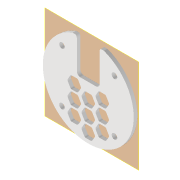
# Autodesk Inventor part: IM_Matchboxscope_base_xiao_lid
Saved by Autodesk Inventor 2022 (Build 260153000, 153)
## iProperties
Created: 2023-04-27
Part Number: IM_Matchboxscope_base_xiao_lid
Material: Generisch
Document SubType Name: Modeling
Designer: diederichbenedict
Density: 1 g/cm^3
Appearance: Vorgabe
Author: diederichbenedict
Autodesk Inventor part; units mm, degrees
ref_plane "YZ Plane" through (0, 0, 0) normal (1, 0, 0) x (0, 1, 0)
ref_plane "XZ Plane" through (0, 0, 0) normal (0, 1, 0) x (-1, 0, 0)
ref_plane "XY Plane" through (0, 0, 0) normal (0, 0, 1) x (1, 0, 0)
ref_plane "Arbeitsebene1" through (0, 0, 0) normal (0, 0, 1) x (1, 0, 0)
sketch "Skizze1" plane through (0, 0, 0) normal (0, 0, 1) x (1, 0, 0)
  line L0 (8.0712, 15) -> (38.0712, 15)
  line L1 (38.0712, 15) -> (38.0712, -15)
  line L2 (38.0712, -15) -> (8.0712, -15)
  line L3 (8.0712, -15) -> (8.0712, 15)
  line L4 (38.0712, 19) -> (8.0712, 19)
  line L5 (4.0712, 15) -> (4.0712, -15)
  line L6 (8.0712, -19) -> (38.0712, -19)
  line L7 (42.0712, -15) -> (42.0712, 15)
  arc A0 (8.0712, 19) -> (4.0712, 15) centre (8.0712, 15) ccw
  arc A1 (42.0712, 15) -> (38.0712, 19) centre (38.0712, 15) ccw
  arc A2 (38.0712, -19) -> (42.0712, -15) centre (38.0712, -15) ccw
  arc A3 (4.0712, -15) -> (8.0712, -19) centre (8.0712, -15) ccw
  line L8 (29.9712, -18.3074) -> (29.9712, -24.4) projected
  circle A4 centre (38.0712, -15) radius 1.4 projected
  circle A5 centre (38.0712, 15) radius 1.4 projected
  line L9 (39.5712, -24.4) -> (29.9712, -24.4) projected
  line L10 (39.5712, -21.1181) -> (39.5712, -24.4) projected
  line L11 (44.1893, -16.5) -> (39.5712, -21.1181) projected
  line L12 (47.4712, -16.5) -> (44.1893, -16.5) projected
  line L13 (47.4712, 16.5) -> (47.4712, -16.5) projected
  line L14 (44.1893, 16.5) -> (47.4712, 16.5) projected
  line L15 (39.5712, 21.1181) -> (44.1893, 16.5) projected
  line L16 (39.5712, 24.4) -> (39.5712, 21.1181) projected
  line L17 (31.5712, 24.4) -> (39.5712, 24.4) projected
  line L18 (31.5712, 4.0068) -> (31.5712, 24.4) projected
  arc A6 (32.7786, 1.7) -> (31.5712, 4.0068) centre (29.9712, 1.7) ccw projected
  line L19 (32.7786, 1.7) -> (32.7786, -15.5) projected
  arc A7 (29.9712, -18.3074) -> (32.7786, -15.5) centre (29.9712, -15.5) ccw projected
  arc A8 (16.5712, 25.149) -> (3.3138, -16.9) centre (23.0897, -0.0206) ccw
  circle A9 centre (23.0897, -0.0206) radius 26
  point P0 (0, 0)
  point P1 (36.5793, -24.4)
  point P2 (31.5712, 11.3758)
  point P3 (3.3138, -16.9)
  dimension "d0" = 4
  dimension "d1" = 4
  constraints: 16 end point, 10 point on circle, 8 tangent, 5 centre point, 4 parallel, 3 equal radius, 2 perpendicular, 1 coincident, 1 horizontal, 10 other
  measures "d0" distance between parallel lines of L0 L4
  measures "d1" radius of A0
extrude "Extrusion1" add sketch "Skizze1" along normal blind 2 contours L3 L2 L19 A7 L8 L6 A3 L5 A0 L4 L18 L0 | L0 L18 A6 L19 L2 L3 | L18 L4 A1 L7 A2 L6 L8 A7 L19 L2 A4 L1 A5 L0 | L0 A5 L1 A4 L2 L19 A6 L18 | A5 L1 L0 | L0 L1 A5 | L18 L17 A9 L13 L9 L8 L6 A2 L7 A1 L4 | L4 A0 L5 A3 L6 L8 L9 A9 A8 L17 L18 | A4 L1 L2 | L2 L1 A4 | A9 L13
ref_plane "Arbeitsebene2" through (0, 0, 0) normal (0, 0, 1) x (1, 0, 0)
sketch "Skizze2" plane through (0, 0, 2) normal (0, 0, 1) x (1, 0, 0)
  arc A0 (8.0712, 19) -> (4.0712, 15) centre (8.0712, 15) ccw projected
  line L0 (4.0712, 15) -> (4.0712, -15) projected
  arc A1 (4.0712, -15) -> (8.0712, -19) centre (8.0712, -15) ccw projected
  line L1 (8.0712, -19) -> (38.0712, -19) projected
  arc A2 (38.0712, -19) -> (42.0712, -15) centre (38.0712, -15) ccw projected
  line L2 (42.0712, -15) -> (42.0712, 15) projected
  arc A3 (42.0712, 15) -> (38.0712, 19) centre (38.0712, 15) ccw projected
  line L3 (38.0712, 19) -> (8.0712, 19) projected
  circle A4 centre (8.0712, 15) radius 1.4 projected
  circle A5 centre (38.0712, 15) radius 1.4 projected
  circle A6 centre (38.0712, -15) radius 1.4 projected
  circle A7 centre (8.0712, -15) radius 1.4 projected
  point P0 (0, 0)
hole "Bohrung1" at (8.0712, 15, 2) at (8.0712, -15, 2) at (38.0712, -15, 2) at (38.0712, 15, 2) direction (0, 0, -1) diameter 3.2 end through all
sketch "Skizze3" plane through (0, 0, 2) normal (0, 0, 1) x (1, 0, 0)
  circle A0 centre (23.0919, -0.0207) radius 4.25 projected
  arc A1 (30.2483, 24.4) -> (29.5712, 22.9) centre (31.5712, 22.9) ccw projected
  line L0 (39.5712, 24.4) -> (30.2483, 24.4) projected
  line L1 (39.5712, 21.1181) -> (39.5712, 24.4) projected
  line L2 (44.1893, 16.5) -> (39.5712, 21.1181) projected
  line L3 (47.4712, 16.5) -> (44.1893, 16.5) projected
  line L4 (47.4712, -16.5) -> (47.4712, 16.5) projected
  line L5 (44.1893, -16.5) -> (47.4712, -16.5) projected
  line L6 (39.5712, -21.1181) -> (44.1893, -16.5) projected
  line L7 (39.5712, -24.4) -> (39.5712, -21.1181) projected
  line L8 (6.6126, -24.4) -> (39.5712, -24.4) projected
  line L9 (6.6126, -21.1595) -> (6.6126, -24.4) projected
  line L10 (1.9531, -16.5) -> (6.6126, -21.1595) projected
  line L11 (-1.3288, -16.5) -> (1.9531, -16.5) projected
  line L12 (-1.3288, 16.5) -> (-1.3288, -16.5) projected
  line L13 (1.9531, 16.5) -> (-1.3288, 16.5) projected
  line L14 (6.5712, 21.1181) -> (1.9531, 16.5) projected
  line L15 (6.5712, 24.4) -> (6.5712, 21.1181) projected
  line L16 (15.894, 24.4) -> (6.5712, 24.4) projected
  arc A2 (16.5712, 22.9) -> (15.894, 24.4) centre (14.5712, 22.9) ccw projected
  line L17 (16.5712, 22.9) -> (16.5712, 6.5074) projected
  arc A3 (16.5712, 6.5074) -> (18.5712, 4.5074) centre (18.5712, 6.5074) ccw projected
  line L18 (18.5712, 4.5074) -> (27.5712, 4.5074) projected
  arc A4 (27.5712, 4.5074) -> (29.5712, 6.5074) centre (27.5712, 6.5074) ccw projected
  line L19 (29.5712, 6.5074) -> (29.5712, 22.9) projected
  circle A5 centre (38.0712, 15) radius 1.4 projected
  circle A6 centre (8.0712, -15) radius 1.4 projected
  circle A7 centre (38.0712, -15) radius 1.4 projected
  circle A8 centre (8.0712, 15) radius 1.4 projected
  line L20 (15.894, 24.4) -> (30.2483, 24.4)
  line L21 (6.5712, 24.4) -> (39.5712, 24.4)
  line L22 (39.5712, 24.4) -> (39.5712, 27.6612)
  line L23 (39.5712, 27.6612) -> (6.5712, 27.6612)
  line L24 (6.5712, 27.6612) -> (6.5712, 24.4)
  point P0 (0, 0)
  constraints: 10 end point, 2 horizontal, 2 parallel, 1 perpendicular
extrude "Extrusion2" cut sketch "Skizze3" against normal blind 10 contours L20 L16 L24 L23 L22 L0 | A1 L19 A4 L18 A3 L17 A2 L20
fillet "Rundung1" [suppressed]
sketch "Skizze4" plane through (0, 0, 2) normal (0, 0, 1) x (1, 0, 0)
  line L0 (32.0136, 24.4) -> (30.2483, 24.4) projected
  arc A0 (30.2483, 24.4) -> (29.5712, 22.9) centre (31.5712, 22.9) ccw projected
  line L1 (29.5712, 22.9) -> (29.5712, 6.5074) projected
  arc A1 (27.5712, 4.5074) -> (29.5712, 6.5074) centre (27.5712, 6.5074) ccw projected
  line L2 (27.5712, 4.5074) -> (18.5712, 4.5074) projected
  arc A2 (16.5712, 6.5074) -> (18.5712, 4.5074) centre (18.5712, 6.5074) ccw projected
  line L3 (16.5712, 6.5074) -> (16.5712, 22.9) projected
  arc A3 (16.5712, 22.9) -> (15.894, 24.4) centre (14.5712, 22.9) ccw projected
  line L4 (15.894, 24.4) -> (14.1659, 24.4) projected
  arc A4 (14.1659, 24.4) -> (32.0136, 24.4) centre (23.0897, -0.0206) ccw projected
  circle A5 centre (38.0712, 15) radius 1.6 projected
  circle A6 centre (8.0712, -15) radius 1.6 projected
  circle A7 centre (8.0712, 15) radius 1.6 projected
  circle A8 centre (38.0712, -15) radius 1.6 projected
  line L5 (19.3598, -3.9564) -> (20.7825, -1.4923)
  line L6 (21.6485, -0.9923) -> (24.4938, -0.9923)
  line L7 (25.3598, -1.4923) -> (26.7825, -3.9564)
  line L8 (26.7825, -4.9564) -> (25.3598, -7.4205)
  line L9 (24.4938, -7.9205) -> (21.6485, -7.9205)
  line L10 (20.7825, -7.4205) -> (19.3598, -4.9564)
  line L11 (27.5712, 4.5074) -> (18.5712, 4.5074) projected
  arc A9 (26.7825, -4.9564) -> (26.7825, -3.9564) centre (25.9165, -4.4564) ccw
  arc A10 (24.4938, -7.9205) -> (25.3598, -7.4205) centre (24.4938, -6.9205) ccw
  arc A11 (20.7825, -7.4205) -> (21.6485, -7.9205) centre (21.6485, -6.9205) ccw
  arc A12 (19.3598, -3.9564) -> (19.3598, -4.9564) centre (20.2259, -4.4564) ccw
  arc A13 (21.6485, -0.9923) -> (20.7825, -1.4923) centre (21.6485, -1.9923) ccw
  arc A14 (25.3598, -1.4923) -> (24.4938, -0.9923) centre (24.4938, -1.9923) ccw
  line L12 (27.3598, 0.0436) -> (28.7825, 2.5077)
  line L13 (29.6485, 3.0077) -> (32.4938, 3.0077)
  line L14 (33.3598, 2.5077) -> (34.7825, 0.0436)
  line L15 (34.7825, -0.9564) -> (33.3598, -3.4205)
  line L16 (32.4938, -3.9205) -> (29.6485, -3.9205)
  line L17 (28.7825, -3.4205) -> (27.3598, -0.9564)
  arc A15 (34.7825, -0.9564) -> (34.7825, 0.0436) centre (33.9165, -0.4564) ccw
  arc A16 (32.4938, -3.9205) -> (33.3598, -3.4205) centre (32.4938, -2.9205) ccw
  arc A17 (28.7825, -3.4205) -> (29.6485, -3.9205) centre (29.6485, -2.9205) ccw
  arc A18 (27.3598, 0.0436) -> (27.3598, -0.9564) centre (28.2259, -0.4564) ccw
  arc A19 (29.6485, 3.0077) -> (28.7825, 2.5077) centre (29.6485, 2.0077) ccw
  arc A20 (33.3598, 2.5077) -> (32.4938, 3.0077) centre (32.4938, 2.0077) ccw
  line L18 (11.3598, 0.0436) -> (12.7825, 2.5077)
  line L19 (13.6485, 3.0077) -> (16.4938, 3.0077)
  line L20 (17.3598, 2.5077) -> (18.7825, 0.0436)
  line L21 (18.7825, -0.9564) -> (17.3598, -3.4205)
  line L22 (16.4938, -3.9205) -> (13.6485, -3.9205)
  line L23 (12.7825, -3.4205) -> (11.3598, -0.9564)
  arc A21 (18.7825, -0.9564) -> (18.7825, 0.0436) centre (17.9165, -0.4564) ccw
  arc A22 (16.4938, -3.9205) -> (17.3598, -3.4205) centre (16.4938, -2.9205) ccw
  arc A23 (12.7825, -3.4205) -> (13.6485, -3.9205) centre (13.6485, -2.9205) ccw
  arc A24 (11.3598, 0.0436) -> (11.3598, -0.9564) centre (12.2259, -0.4564) ccw
  arc A25 (13.6485, 3.0077) -> (12.7825, 2.5077) centre (13.6485, 2.0077) ccw
  arc A26 (17.3598, 2.5077) -> (16.4938, 3.0077) centre (16.4938, 2.0077) ccw
  point P0 (0, 0)
  point P1 (23.0712, -4.4564)
  point P2 (19.0712, -4.4564)
  point P3 (21.0712, -0.9923)
  point P4 (25.0712, -0.9923)
  point P5 (27.0712, -4.4564)
  point P6 (25.0712, -7.9205)
  point P7 (21.0712, -7.9205)
  point P8 (31.0712, -0.4564)
  point P9 (27.0712, -0.4564)
  point P10 (29.0712, 3.0077)
  point P11 (33.0712, 3.0077)
  point P12 (35.0712, -0.4564)
  point P13 (33.0712, -3.9205)
  point P14 (29.0712, -3.9205)
  point P15 (15.0712, -0.4564)
  point P16 (11.0712, -0.4564)
  point P17 (13.0712, 3.0077)
  point P18 (17.0712, 3.0077)
  point P19 (19.0712, -0.4564)
  point P20 (17.0712, -3.9205)
  point P21 (13.0712, -3.9205)
  dimension "d38" = 8
  dimension "d39" = 1
  dimension "d40" = 8
  dimension "d41" = 1
  dimension "d42" = 8
  dimension "d43" = 1
  dimension "d44" = 4
  dimension "d45" = 8
  dimension "d46" = 4
  dimension "d47" = 8
  dimension "d48" = 13
  dimension "d49" = 6.5
  constraints: 36 end point, 36 point on circle, 36 point on line, 36 tangent, 18 centre point, 15 equal radius, 1 parallel, 39 other
  measures "d38" distance of point (19.071, -4.456) point (27.071, -4.456)
  measures "d39" radius of A9
  measures "d40" distance of point (27.071, -0.456) point (35.071, -0.456)
  measures "d41" radius of A15
  measures "d42" distance of point (11.071, -0.456) point (19.071, -0.456)
  measures "d43" radius of A21
  measures "d44" vertical distance of point (23.071, -4.456) point (31.071, -0.456)
  measures "d45" horizontal distance of point (23.071, -4.456) point (31.071, -0.456)
  measures "d46" vertical distance of point (23.071, -4.456) point (15.071, -0.456)
  measures "d47" horizontal distance of point (15.071, -0.456) point (23.071, -4.456)
  measures "d48" distance between parallel lines of L3 L1
  measures "d49" distance from line of point (23.071, -4.456) L1
extrude "Extrusion3" cut sketch "Skizze4" against normal blind 4 contours L5 A13 L6 A14 L7 A9 L8 A10 L9 A11 L10 A12 | L12 A19 L13 A20 L14 A15 L15 A16 L16 A17 L17 A18 | L18 A25 L19 A26 L20 A21 L21 A22 L22 A23 L23 A24
pattern_linear "Rechteckige Anordnung1" count 3 spacing 8 along (0, -1, 0) of "Extrusion3"
equation "\"d27\" = d44"
